Autodesk Fusion 360 part; units mm, degrees
(part 3 of 4)
sketch "Sketch9" plane through (0, 0, 1.5) normal (0, 0, 1) x (-1, 0, 0)
  ellipse E0 centre (-56, -51.25) end of major axis (-52, -51.25) minor radius 1 (-56, -52.25) -> (-56, -50.25) ccw
  line L0 (-56, -52.25) -> (-74.75, -52.25)
  ellipse E1 centre (-74.75, -51.25) end of major axis (-70.75, -51.25) minor radius 1 (-74.75, -50.25) -> (-74.75, -52.25) ccw
  line L1 (-74.75, -50.25) -> (-56, -50.25)
  ellipse E2 centre (-74.75, -23.25) end of major axis (-70.75, -23.25) minor radius 1 (-74.75, -22.25) -> (-74.75, -24.25) ccw
  line L2 (-74.75, -22.25) -> (-56, -22.25)
  ellipse E3 centre (-56, -23.25) end of major axis (-52, -23.25) minor radius 1 (-56, -24.25) -> (-56, -22.25) ccw
  line L3 (-56, -24.25) -> (-74.75, -24.25)
  ellipse E4 centre (-38, -30.25) end of major axis (-34, -30.25) minor radius 1 (-38, -29.25) -> (-38, -31.25) ccw
  line L4 (-38, -29.25) -> (-19.25, -29.25)
  ellipse E5 centre (-19.25, -30.25) end of major axis (-15.25, -30.25) minor radius 1 (-19.25, -31.25) -> (-19.25, -29.25) ccw
  line L5 (-19.25, -31.25) -> (-38, -31.25)
  ellipse E6 centre (-38, -58.25) end of major axis (-34, -58.25) minor radius 1 (-38, -57.25) -> (-38, -59.25) ccw
  line L6 (-38, -57.25) -> (-19.25, -57.25)
  ellipse E7 centre (-19.25, -58.25) end of major axis (-15.25, -58.25) minor radius 1 (-19.25, -59.25) -> (-19.25, -57.25) ccw
  line L7 (-19.25, -59.25) -> (-38, -59.25)
  ellipse E8 centre (-19.25, -51.25) end of major axis (-15.25, -51.25) minor radius 1 (-19.25, -52.25) -> (-19.25, -50.25) ccw
  line L8 (-19.25, -52.25) -> (-38, -52.25)
  ellipse E9 centre (-38, -51.25) end of major axis (-34, -51.25) minor radius 1 (-38, -50.25) -> (-38, -52.25) ccw
  line L9 (-38, -50.25) -> (-19.25, -50.25)
  ellipse E10 centre (-19.25, -23.25) end of major axis (-15.25, -23.25) minor radius 1 (-19.25, -24.25) -> (-19.25, -22.25) ccw
  line L10 (-19.25, -24.25) -> (-38, -24.25)
  ellipse E11 centre (-38, -23.25) end of major axis (-34, -23.25) minor radius 1 (-38, -22.25) -> (-38, -24.25) ccw
  line L11 (-38, -22.25) -> (-19.25, -22.25)
  ellipse E12 centre (-74.75, -30.25) end of major axis (-70.75, -30.25) minor radius 1 (-74.75, -29.25) -> (-74.75, -31.25) ccw
  line L12 (-74.75, -29.25) -> (-56, -29.25)
  ellipse E13 centre (-56, -30.25) end of major axis (-52, -30.25) minor radius 1 (-56, -31.25) -> (-56, -29.25) ccw
  line L13 (-56, -31.25) -> (-74.75, -31.25)
  ellipse E14 centre (-74.75, -58.25) end of major axis (-70.75, -58.25) minor radius 1 (-74.75, -57.25) -> (-74.75, -59.25) ccw
  line L14 (-74.75, -57.25) -> (-56, -57.25)
  ellipse E15 centre (-56, -58.25) end of major axis (-52, -58.25) minor radius 1 (-56, -59.25) -> (-56, -57.25) ccw
  line L15 (-56, -59.25) -> (-74.75, -59.25)
  ellipse E16 centre (-74.75, -44.25) end of major axis (-70.75, -44.25) minor radius 1 (-74.75, -43.25) -> (-74.75, -45.25) ccw
  line L16 (-74.75, -43.25) -> (-56, -43.25)
  ellipse E17 centre (-56, -44.25) end of major axis (-52, -44.25) minor radius 1 (-56, -45.25) -> (-56, -43.25) ccw
  line L17 (-56, -45.25) -> (-74.75, -45.25)
  ellipse E18 centre (-74.75, -16.25) end of major axis (-70.75, -16.25) minor radius 1 (-74.75, -15.25) -> (-74.75, -17.25) ccw
  line L18 (-74.75, -15.25) -> (-56, -15.25)
  ellipse E19 centre (-56, -16.25) end of major axis (-52, -16.25) minor radius 1 (-56, -17.25) -> (-56, -15.25) ccw
  line L19 (-56, -17.25) -> (-74.75, -17.25)
  ellipse E20 centre (-19.25, -37.25) end of major axis (-15.25, -37.25) minor radius 1 (-19.25, -38.25) -> (-19.25, -36.25) ccw
  line L20 (-19.25, -38.25) -> (-38, -38.25)
  ellipse E21 centre (-38, -37.25) end of major axis (-34, -37.25) minor radius 1 (-38, -36.25) -> (-38, -38.25) ccw
  line L21 (-38, -36.25) -> (-19.25, -36.25)
  ellipse E22 centre (-19.25, -65.25) end of major axis (-15.25, -65.25) minor radius 1 (-19.25, -66.25) -> (-19.25, -64.25) ccw
  line L22 (-19.25, -66.25) -> (-38, -66.25)
  ellipse E23 centre (-38, -65.25) end of major axis (-34, -65.25) minor radius 1 (-38, -64.25) -> (-38, -66.25) ccw
  line L23 (-38, -64.25) -> (-19.25, -64.25)
  ellipse E24 centre (-38, -44.25) end of major axis (-34, -44.25) minor radius 1 (-38, -43.25) -> (-38, -45.25) ccw
  line L24 (-38, -43.25) -> (-19.25, -43.25)
  ellipse E25 centre (-19.25, -44.25) end of major axis (-15.25, -44.25) minor radius 1 (-19.25, -45.25) -> (-19.25, -43.25) ccw
  line L25 (-19.25, -45.25) -> (-38, -45.25)
  ellipse E26 centre (-38, -16.25) end of major axis (-34, -16.25) minor radius 1 (-38, -15.25) -> (-38, -17.25) ccw
  line L26 (-38, -15.25) -> (-19.25, -15.25)
  ellipse E27 centre (-19.25, -16.25) end of major axis (-15.25, -16.25) minor radius 1 (-19.25, -17.25) -> (-19.25, -15.25) ccw
  line L27 (-19.25, -17.25) -> (-38, -17.25)
  line L28 (-74.75, -36.25) -> (-56, -36.25)
  ellipse E28 centre (-56, -37.25) end of major axis (-52, -37.25) minor radius 1 (-56, -38.25) -> (-56, -36.25) ccw
  line L29 (-56, -38.25) -> (-74.75, -38.25)
  ellipse E29 centre (-74.75, -37.25) end of major axis (-70.75, -37.25) minor radius 1 (-74.75, -36.25) -> (-74.75, -38.25) ccw
  ellipse E30 centre (-74.75, -65.25) end of major axis (-70.75, -65.25) minor radius 1 (-74.75, -64.25) -> (-74.75, -66.25) ccw
  line L30 (-74.75, -64.25) -> (-56, -64.25)
  ellipse E31 centre (-56, -65.25) end of major axis (-52, -65.25) minor radius 1 (-56, -66.25) -> (-56, -64.25) ccw
  line L31 (-56, -66.25) -> (-74.75, -66.25)
  line L32 (-34.7574, -85.9106) -> (-28.1106, -92.5574)
  ellipse E32 centre (-28.8177, -93.2645) end of major axis (-25.9892, -96.0929) minor radius 1 (-29.5248, -93.9716) -> (-28.1106, -92.5574) ccw
  line L33 (-29.5248, -93.9716) -> (-36.1716, -87.3248)
  ellipse E33 centre (-35.4645, -86.6177) end of major axis (-32.636, -89.4461) minor radius 1 (-34.7574, -85.9106) -> (-36.1716, -87.3248) ccw
  ellipse E34 centre (-73.5355, -93.2645) end of major axis (-70.7071, -90.436) minor radius 1 (-74.2426, -92.5574) -> (-72.8284, -93.9716) ccw
  line L34 (-74.2426, -92.5574) -> (-56.8095, -75.1242)
  ellipse E35 centre (-56.1024, -75.8313) end of major axis (-53.2739, -73.0029) minor radius 1 (-55.3953, -76.5384) -> (-56.8095, -75.1242) ccw
  line L35 (-55.3953, -76.5384) -> (-72.8284, -93.9716)
  ellipse E36 centre (-38.4645, -75.7892) end of major axis (-35.636, -78.6177) minor radius 1 (-37.7574, -75.0821) -> (-39.1716, -76.4963) ccw
  line L36 (-37.7574, -75.0821) -> (-20.2821, -92.5574)
  ellipse E37 centre (-20.9892, -93.2645) end of major axis (-18.1608, -96.0929) minor radius 1 (-21.6963, -93.9716) -> (-20.2821, -92.5574) ccw
  line L37 (-21.6963, -93.9716) -> (-39.1716, -76.4963)
  ellipse E38 centre (-58.5355, -93.9213) end of major axis (-55.7071, -91.0929) minor radius 1 (-57.5048, -94.2952) -> (-58.9094, -92.8906) ccw
  ellipse E39 centre (-57.8787, -93.2645) end of major axis (-55.0503, -90.436) minor radius 1 (-58.9094, -92.8906) -> (-57.5048, -94.2952) ccw
  ellipse E40 centre (-65.7071, -93.2645) end of major axis (-62.8787, -90.436) minor radius 1 (-66.4142, -92.5574) -> (-65, -93.9716) ccw
  line L38 (-66.4142, -92.5574) -> (-59.2426, -85.3858)
  ellipse E41 centre (-58.5355, -86.0929) end of major axis (-55.7071, -83.2645) minor radius 1 (-57.8284, -86.8) -> (-59.2426, -85.3858) ccw
  line L39 (-57.8284, -86.8) -> (-65, -93.9716)
  ellipse E42 centre (-35.6289, -93.7569) end of major axis (-32.8005, -96.5853) minor radius 1 (-35.1707, -92.8062) -> (-36.5796, -94.2151) ccw
  ellipse E43 centre (-36.1213, -93.2645) end of major axis (-33.2929, -96.0929) minor radius 1 (-36.5796, -94.2151) -> (-35.1707, -92.8062) ccw
  line L40 (-93.75, -111.8) -> (-0.25, -111.8)
  line L41 (-0.25, -111.8) -> (-0.25, -0.25)
  line L42 (-0.25, -0.25) -> (-93.75, -0.25)
  line L43 (-93.75, -0.25) -> (-93.75, -111.8)
  circle A0 centre (-5, -5) radius 2
  circle A1 centre (-3.5, -95.55) radius 2
  circle A2 centre (-90.5, -95.55) radius 2
  circle A3 centre (-87.5, -6.5) radius 2
  line L44 (-42.5, -83.8) -> (-42.5, -96.8)
  line L45 (-42.5, -96.8) -> (-51.5, -96.8)
  line L46 (-51.5, -96.8) -> (-51.5, -83.8)
  line L47 (-51.5, -83.8) -> (-42.5, -83.8)
  line L48 (-42, -100.3) -> (-42, -110.3)
  line L49 (-42, -110.3) -> (-43.9689, -110.3)
  line L50 (-43.9689, -110.3) -> (-43.9689, -103.55)
  line L51 (-43.9689, -103.55) -> (-47, -101.8)
  line L52 (-47, -101.8) -> (-50.0311, -103.55)
  line L53 (-50.0311, -103.55) -> (-50.0311, -110.3)
  line L54 (-50.0311, -110.3) -> (-52, -110.3)
  line L55 (-52, -110.3) -> (-52, -100.3)
  line L56 (-52, -100.3) -> (-55, -100.3)
  line L57 (-55, -100.3) -> (-55, -80.3)
  line L58 (-55, -80.3) -> (-52, -80.3)
  line L59 (-52, -80.3) -> (-52, -81.8)
  line L60 (-52, -81.8) -> (-53.5, -81.8)
  line L61 (-53.5, -81.8) -> (-53.5, -98.8)
  line L62 (-53.5, -98.8) -> (-40.5, -98.8)
  line L63 (-40.5, -98.8) -> (-40.5, -81.8)
  line L64 (-40.5, -81.8) -> (-42, -81.8)
  line L65 (-42, -81.8) -> (-42, -80.3)
  line L66 (-42, -80.3) -> (-39, -80.3)
  line L67 (-39, -80.3) -> (-39, -100.3)
  line L68 (-39, -100.3) -> (-42, -100.3)
  line L69 (-0.25, -111.8) -> (-15.25, -111.8)
  line L70 (-15.25, -111.8) -> (-15.25, -96.8)
  line L71 (-15.25, -96.8) -> (-0.25, -96.8)
  line L72 (-0.25, -96.8) -> (-0.25, -111.8)
  line L73 (-93.75, -0.25) -> (-78.75, -0.25)
  line L74 (-78.75, -0.25) -> (-78.75, -15.25)
  line L75 (-78.75, -15.25) -> (-93.75, -15.25)
  line L76 (-93.75, -15.25) -> (-93.75, -0.25)
  line L77 (-15.25, -96.8) -> (-78.75, -96.8)
  line L78 (-78.75, -96.8) -> (-78.75, -15.25)
  line L79 (-78.75, -15.25) -> (-15.25, -15.25)
  line L80 (-15.25, -15.25) -> (-15.25, -96.8)
  line L81 (-47, -96.8) -> (-42, -96.8)
  line L82 (-42, -96.8) -> (-42, -15.25)
  line L83 (-42, -15.25) -> (-47, -15.25)
  line L84 (-47, -15.25) -> (-47, -96.8)
  line L85 (-47, -96.8) -> (-52, -96.8)
  line L86 (-52, -96.8) -> (-52, -15.25)
  line L87 (-52, -15.25) -> (-47, -15.25)
  line L88 (-47, -15.25) -> (-47, -96.8)
  line L89 (-28.625, -66.25) -> (-42, -66.25)
  line L90 (-28.625, -66.25) -> (-15.25, -66.25)
  line L91 (-15.25, -66.25) -> (-78.75, -66.25)
  line L92 (-29.0197, -83.8197) -> (-16.0395, -96.8)
  line L93 (-16.0395, -96.8) -> (-11.0395, -96.8)
  line L94 (-29.2885, -83.551) -> (-29.0197, -83.8197)
  line L95 (-29.0197, -83.8197) -> (-42, -70.8395)
  line L96 (-42, -70.8395) -> (-42, -68.8395)
  line L97 (-42, -68.8395) -> (-15.25, -84.2836)
  line L98 (-42, -68.8395) -> (-11.1118, -68.8395) construction
  line L99 (-42, -68.8395) -> (-41, -67.1074)
  line L100 (-41, -67.1074) -> (-15.25, -81.9742)
  line L101 (-15.25, -81.9742) -> (-16.25, -83.7063)
  line L102 (-16.25, -83.7063) -> (-19.7141, -81.7063)
  line L103 (-19.7141, -81.7063) -> (-18.7141, -79.9742)
  line L104 (-42, -68.8395) -> (-38.5359, -70.8395)
  line L105 (-38.5359, -70.8395) -> (-37.5359, -69.1074)
  line L106 (-42, -68.8395) -> (-52, -68.8395)
  line L107 (-52, -68.8395) -> (-78.75, -84.2836)
  line L108 (-52, -68.8395) -> (-53, -67.1074)
  line L109 (-53, -67.1074) -> (-78.75, -81.9742)
  line L110 (-78.75, -81.9742) -> (-77.75, -83.7063)
  line L111 (-52, -68.8395) -> (-55.4641, -70.8395)
  line L112 (-55.4641, -70.8395) -> (-56.4641, -69.1074)
  line L113 (-55.4641, -70.8395) -> (-53.4641, -70.8395) construction
  line L114 (-77.75, -83.7063) -> (-74.2859, -81.7063)
  line L115 (-74.2859, -81.7063) -> (-75.2859, -79.9742)
  ellipse E44 centre (-19.2141, -80.8402) end of major axis (-19.7141, -81.7063) minor radius 4
  line L116 (-18.7141, -79.9742) -> (-19.7141, -81.7063)
  line L117 (-22.6782, -78.8402) -> (-15.75, -82.8402)
  ellipse E45 centre (-38.0359, -69.9735) end of major axis (-38.5359, -70.8395) minor radius 4
  line L118 (-37.5359, -69.1074) -> (-38.5359, -70.8395)
  line L119 (-41.5, -67.9735) -> (-34.5718, -71.9735)
  ellipse E46 centre (-55.9641, -69.9735) end of major axis (-55.4641, -70.8395) minor radius 4
  line L120 (-56.4641, -69.1074) -> (-55.4641, -70.8395)
  line L121 (-59.4282, -71.9735) -> (-52.5, -67.9735)
  ellipse E47 centre (-74.7859, -80.8402) end of major axis (-74.2859, -81.7063) minor radius 4
  line L122 (-75.2859, -79.9742) -> (-74.2859, -81.7063)
  line L123 (-78.25, -82.8402) -> (-71.3218, -78.8402)
  dimension "d217" = 15
  dimension "d218" = 15
  dimension "d219" = 15
  dimension "d220" = 15
  dimension "d221" = 5
  dimension "d222" = 5
  dimension "d223" = 5
  dimension "d224" = 2
  dimension "d225" = 30
  dimension "d226" = 2
  dimension "d227" = 4
  dimension "d228" = 4
  dimension "d229" = 30
  dimension "d230" = 90
  dimension "d231" = 2
  dimension "d232" = 4
  dimension "d233" = 120
  dimension "d234" = 4
  constraint horizontal L69
  constraint vertical L70
  constraint horizontal L71
  constraint vertical L72
  constraint coincident L40.end L41.start
  constraint horizontal L73
  constraint vertical L74
  constraint horizontal L75
  constraint vertical L76
  constraint coincident L42.end L43.start
  constraint horizontal L77
  constraint vertical L78
  constraint horizontal L79
  constraint vertical L80
  constraint horizontal L81
  constraint vertical L82
  constraint horizontal L83
  constraint vertical L84
  constraint coincident L79 L82.end
  constraint midpoint L45 L81.start
  constraint horizontal L85
  constraint vertical L86
  constraint horizontal L87
  constraint vertical L88
  constraint midpoint L22 L89.start
  constraint coincident L82 L89.end
  constraint perpendicular L82 L89
  constraint coincident L80 L90.end
  constraint perpendicular L80 L90
  constraint coincident L78 L91.end
  constraint perpendicular L78 L91
  constraint midpoint L36 L92.start
  constraint coincident L77 L92.end
  constraint parallel L36 L92
  constraint perpendicular L70 L93
  constraint coincident L36 L94.start
  constraint parallel L92 L94
  constraint coincident L82 L95.end
  constraint parallel L36 L95
  constraint parallel L82 L96
  constraint horizontal L98
  constraint coincident L80 L97.end
  constraint perpendicular L97 L99
  constraint coincident L80 L100.end
  constraint perpendicular L99 L100
  constraint coincident L97 L101.end
  constraint perpendicular L97 L101
  constraint perpendicular L101 L102
  constraint coincident L100 L103.end
  constraint perpendicular L100 L103
  constraint perpendicular L99 L104
  constraint coincident L100 L105.end
  constraint perpendicular L100 L105
  constraint coincident L86 L106.end
  constraint perpendicular L86 L106
  constraint coincident L78 L107.end
  constraint coincident L78 L109.end
  constraint perpendicular L108 L109
  constraint coincident L107 L110.end
  constraint perpendicular L107 L110
  constraint perpendicular L110 L111
  constraint horizontal L113
  constraint coincident L109 L112.end
  constraint perpendicular L110 L114
  constraint coincident L109 L115.end
  constraint perpendicular L109 L115
  constraint midpoint L103 E44.centre
  constraint coincident L103.end E44
  constraint coincident L102.end E44
  constraint midpoint L105 E45.centre
  constraint coincident L105.end E45
  constraint coincident L104.end E45
  constraint midpoint L112 E46.centre
  constraint coincident L112.end E46
  constraint coincident L111.end E46
  constraint midpoint L115 E47.centre
  constraint coincident L115.end E47
  constraint coincident L114.end E47
  measures "d217" distance of L40.end L69.end
  measures "d218" distance of L40.end L71.end
  measures "d219" distance of L42.end L73.end
  measures "d220" distance of L42.end L75.end
  measures "d221" distance of L81.start L81.end
  measures "d222" distance of L81.start L85.end
  measures "d223" distance of L92.end L93.end
  measures "d224" distance of L95.end L96.end
  measures "d225" angle of L97 L98
  measures "d226" distance of L96.end L99.end
  measures "d227" distance of L101.end L102.end
  measures "d228" distance of L96.end L104.end
  measures "d229" angle of L106 L107
  measures "d230" angle of L107 L108
  measures "d231" distance of L106.end L108.end
  measures "d232" distance of L106.end L111.end
  measures "d233" angle of L112 L113
  measures "d234" distance of L110.end L114.end
extrude "Extrude13" cut sketch "Sketch9" against normal blind 4 contours L112 E46 L120 L121 | L107 L109 E46 E47 | L112 E46 L120 L121 | L112 E46 L120 L121 | L115 E47 L122 L123 | L115 E47 L122 L123 | L112 E46 L120 L121 | L115 E47 L122 L123 | L115 E47 L122 L123 | L97 L100 E44 E45 | L105 E45 L118 L119 | L105 E45 L118 L119 | L105 E45 L118 L119 | L103 E44 L116 L117 | L103 E44 L116 L117 | L105 E45 L118 L119 | L103 E44 L116 L117 | L103 E44 L116 L117
sketch "Sketch10" plane through (0, 0, 1.5) normal (0, 0, 1) x (-1, 0, 0)
  ellipse E0 centre (-19.2141, -80.8402) end of major axis (-15.75, -82.8402) minor radius 1 (-19.7141, -81.7063) -> (-18.7141, -79.9742) ccw
  line L0 (-19.7141, -81.7063) -> (-38.5359, -70.8395)
  ellipse E1 centre (-38.0359, -69.9735) end of major axis (-34.5718, -71.9735) minor radius 1 (-37.5359, -69.1074) -> (-38.5359, -70.8395) ccw
  line L1 (-37.5359, -69.1074) -> (-18.7141, -79.9742)
  ellipse E2 centre (-74.7859, -80.8402) end of major axis (-71.3218, -78.8402) minor radius 1 (-75.2859, -79.9742) -> (-74.2859, -81.7063) ccw
  line L2 (-75.2859, -79.9742) -> (-56.4641, -69.1074)
  ellipse E3 centre (-55.9641, -69.9735) end of major axis (-52.5, -67.9735) minor radius 1 (-55.4641, -70.8395) -> (-56.4641, -69.1074) ccw
  line L3 (-55.4641, -70.8395) -> (-74.2859, -81.7063)
  ellipse E4 centre (-56, -51.25) end of major axis (-52, -51.25) minor radius 1 (-56, -52.25) -> (-56, -50.25) ccw
  line L4 (-56, -52.25) -> (-74.75, -52.25)
  ellipse E5 centre (-74.75, -51.25) end of major axis (-70.75, -51.25) minor radius 1 (-74.75, -50.25) -> (-74.75, -52.25) ccw
  line L5 (-74.75, -50.25) -> (-56, -50.25)
  ellipse E6 centre (-74.75, -23.25) end of major axis (-70.75, -23.25) minor radius 1 (-74.75, -22.25) -> (-74.75, -24.25) ccw
  line L6 (-74.75, -22.25) -> (-56, -22.25)
  ellipse E7 centre (-56, -23.25) end of major axis (-52, -23.25) minor radius 1 (-56, -24.25) -> (-56, -22.25) ccw
  line L7 (-56, -24.25) -> (-74.75, -24.25)
  ellipse E8 centre (-38, -30.25) end of major axis (-34, -30.25) minor radius 1 (-38, -29.25) -> (-38, -31.25) ccw
  line L8 (-38, -29.25) -> (-19.25, -29.25)
  ellipse E9 centre (-19.25, -30.25) end of major axis (-15.25, -30.25) minor radius 1 (-19.25, -31.25) -> (-19.25, -29.25) ccw
  line L9 (-19.25, -31.25) -> (-38, -31.25)
  ellipse E10 centre (-38, -58.25) end of major axis (-34, -58.25) minor radius 1 (-38, -57.25) -> (-38, -59.25) ccw
  line L10 (-38, -57.25) -> (-19.25, -57.25)
  ellipse E11 centre (-19.25, -58.25) end of major axis (-15.25, -58.25) minor radius 1 (-19.25, -59.25) -> (-19.25, -57.25) ccw
  line L11 (-19.25, -59.25) -> (-38, -59.25)
  ellipse E12 centre (-19.25, -51.25) end of major axis (-15.25, -51.25) minor radius 1 (-19.25, -52.25) -> (-19.25, -50.25) ccw
  line L12 (-19.25, -52.25) -> (-38, -52.25)
  ellipse E13 centre (-38, -51.25) end of major axis (-34, -51.25) minor radius 1 (-38, -50.25) -> (-38, -52.25) ccw
  line L13 (-38, -50.25) -> (-19.25, -50.25)
  ellipse E14 centre (-19.25, -23.25) end of major axis (-15.25, -23.25) minor radius 1 (-19.25, -24.25) -> (-19.25, -22.25) ccw
  line L14 (-19.25, -24.25) -> (-38, -24.25)
  ellipse E15 centre (-38, -23.25) end of major axis (-34, -23.25) minor radius 1 (-38, -22.25) -> (-38, -24.25) ccw
  line L15 (-38, -22.25) -> (-19.25, -22.25)
  ellipse E16 centre (-74.75, -30.25) end of major axis (-70.75, -30.25) minor radius 1 (-74.75, -29.25) -> (-74.75, -31.25) ccw
  line L16 (-74.75, -29.25) -> (-56, -29.25)
  ellipse E17 centre (-56, -30.25) end of major axis (-52, -30.25) minor radius 1 (-56, -31.25) -> (-56, -29.25) ccw
  line L17 (-56, -31.25) -> (-74.75, -31.25)
  ellipse E18 centre (-74.75, -58.25) end of major axis (-70.75, -58.25) minor radius 1 (-74.75, -57.25) -> (-74.75, -59.25) ccw
  line L18 (-74.75, -57.25) -> (-56, -57.25)
  ellipse E19 centre (-56, -58.25) end of major axis (-52, -58.25) minor radius 1 (-56, -59.25) -> (-56, -57.25) ccw
  line L19 (-56, -59.25) -> (-74.75, -59.25)
  ellipse E20 centre (-74.75, -44.25) end of major axis (-70.75, -44.25) minor radius 1 (-74.75, -43.25) -> (-74.75, -45.25) ccw
  line L20 (-74.75, -43.25) -> (-56, -43.25)
  ellipse E21 centre (-56, -44.25) end of major axis (-52, -44.25) minor radius 1 (-56, -45.25) -> (-56, -43.25) ccw
  line L21 (-56, -45.25) -> (-74.75, -45.25)
  ellipse E22 centre (-74.75, -16.25) end of major axis (-70.75, -16.25) minor radius 1 (-74.75, -15.25) -> (-74.75, -17.25) ccw
  line L22 (-74.75, -15.25) -> (-56, -15.25)
  ellipse E23 centre (-56, -16.25) end of major axis (-52, -16.25) minor radius 1 (-56, -17.25) -> (-56, -15.25) ccw
  line L23 (-56, -17.25) -> (-74.75, -17.25)
  ellipse E24 centre (-19.25, -37.25) end of major axis (-15.25, -37.25) minor radius 1 (-19.25, -38.25) -> (-19.25, -36.25) ccw
  line L24 (-19.25, -38.25) -> (-38, -38.25)
  ellipse E25 centre (-38, -37.25) end of major axis (-34, -37.25) minor radius 1 (-38, -36.25) -> (-38, -38.25) ccw
  line L25 (-38, -36.25) -> (-19.25, -36.25)
  ellipse E26 centre (-19.25, -65.25) end of major axis (-15.25, -65.25) minor radius 1 (-19.25, -66.25) -> (-19.25, -64.25) ccw
  line L26 (-19.25, -66.25) -> (-38, -66.25)
  ellipse E27 centre (-38, -65.25) end of major axis (-34, -65.25) minor radius 1 (-38, -64.25) -> (-38, -66.25) ccw
  line L27 (-38, -64.25) -> (-19.25, -64.25)
  ellipse E28 centre (-38, -44.25) end of major axis (-34, -44.25) minor radius 1 (-38, -43.25) -> (-38, -45.25) ccw
  line L28 (-38, -43.25) -> (-19.25, -43.25)
  ellipse E29 centre (-19.25, -44.25) end of major axis (-15.25, -44.25) minor radius 1 (-19.25, -45.25) -> (-19.25, -43.25) ccw
  line L29 (-19.25, -45.25) -> (-38, -45.25)
  ellipse E30 centre (-38, -16.25) end of major axis (-34, -16.25) minor radius 1 (-38, -15.25) -> (-38, -17.25) ccw
  line L30 (-38, -15.25) -> (-19.25, -15.25)
  ellipse E31 centre (-19.25, -16.25) end of major axis (-15.25, -16.25) minor radius 1 (-19.25, -17.25) -> (-19.25, -15.25) ccw
  line L31 (-19.25, -17.25) -> (-38, -17.25)
  line L32 (-74.75, -36.25) -> (-56, -36.25)
  ellipse E32 centre (-56, -37.25) end of major axis (-52, -37.25) minor radius 1 (-56, -38.25) -> (-56, -36.25) ccw
  line L33 (-56, -38.25) -> (-74.75, -38.25)
  ellipse E33 centre (-74.75, -37.25) end of major axis (-70.75, -37.25) minor radius 1 (-74.75, -36.25) -> (-74.75, -38.25) ccw
  ellipse E34 centre (-74.75, -65.25) end of major axis (-70.75, -65.25) minor radius 1 (-74.75, -64.25) -> (-74.75, -66.25) ccw
  line L34 (-74.75, -64.25) -> (-56, -64.25)
  ellipse E35 centre (-56, -65.25) end of major axis (-52, -65.25) minor radius 1 (-56, -66.25) -> (-56, -64.25) ccw
  line L35 (-56, -66.25) -> (-74.75, -66.25)
  line L36 (-34.7574, -85.9106) -> (-28.1106, -92.5574)
  ellipse E36 centre (-28.8177, -93.2645) end of major axis (-25.9892, -96.0929) minor radius 1 (-29.5248, -93.9716) -> (-28.1106, -92.5574) ccw
  line L37 (-29.5248, -93.9716) -> (-36.1716, -87.3248)
  ellipse E37 centre (-35.4645, -86.6177) end of major axis (-32.636, -89.4461) minor radius 1 (-34.7574, -85.9106) -> (-36.1716, -87.3248) ccw
  ellipse E38 centre (-73.5355, -93.2645) end of major axis (-70.7071, -90.436) minor radius 1 (-74.2426, -92.5574) -> (-72.8284, -93.9716) ccw
  line L38 (-74.2426, -92.5574) -> (-56.8095, -75.1242)
  ellipse E39 centre (-56.1024, -75.8313) end of major axis (-53.2739, -73.0029) minor radius 1 (-55.3953, -76.5384) -> (-56.8095, -75.1242) ccw
  line L39 (-55.3953, -76.5384) -> (-72.8284, -93.9716)
  ellipse E40 centre (-38.4645, -75.7892) end of major axis (-35.636, -78.6177) minor radius 1 (-37.7574, -75.0821) -> (-39.1716, -76.4963) ccw
  line L40 (-37.7574, -75.0821) -> (-20.2821, -92.5574)
  ellipse E41 centre (-20.9892, -93.2645) end of major axis (-18.1608, -96.0929) minor radius 1 (-21.6963, -93.9716) -> (-20.2821, -92.5574) ccw
  line L41 (-21.6963, -93.9716) -> (-39.1716, -76.4963)
  ellipse E42 centre (-58.5355, -93.9213) end of major axis (-55.7071, -91.0929) minor radius 1 (-57.5048, -94.2952) -> (-58.9094, -92.8906) ccw
  ellipse E43 centre (-57.8787, -93.2645) end of major axis (-55.0503, -90.436) minor radius 1 (-58.9094, -92.8906) -> (-57.5048, -94.2952) ccw
  ellipse E44 centre (-65.7071, -93.2645) end of major axis (-62.8787, -90.436) minor radius 1 (-66.4142, -92.5574) -> (-65, -93.9716) ccw
  line L42 (-66.4142, -92.5574) -> (-59.2426, -85.3858)
  ellipse E45 centre (-58.5355, -86.0929) end of major axis (-55.7071, -83.2645) minor radius 1 (-57.8284, -86.8) -> (-59.2426, -85.3858) ccw
  line L43 (-57.8284, -86.8) -> (-65, -93.9716)
  ellipse E46 centre (-35.6289, -93.7569) end of major axis (-32.8005, -96.5853) minor radius 1 (-35.1707, -92.8062) -> (-36.5796, -94.2151) ccw
  ellipse E47 centre (-36.1213, -93.2645) end of major axis (-33.2929, -96.0929) minor radius 1 (-36.5796, -94.2151) -> (-35.1707, -92.8062) ccw
  line L44 (-93.75, -111.8) -> (-0.25, -111.8)
  line L45 (-0.25, -111.8) -> (-0.25, -0.25)
  line L46 (-0.25, -0.25) -> (-93.75, -0.25)
  line L47 (-93.75, -0.25) -> (-93.75, -111.8)
  circle A0 centre (-5, -5) radius 2
  circle A1 centre (-3.5, -95.55) radius 2
  circle A2 centre (-90.5, -95.55) radius 2
  circle A3 centre (-87.5, -6.5) radius 2
  line L48 (-42.5, -83.8) -> (-42.5, -96.8)
  line L49 (-42.5, -96.8) -> (-51.5, -96.8)
  line L50 (-51.5, -96.8) -> (-51.5, -83.8)
  line L51 (-51.5, -83.8) -> (-42.5, -83.8)
  line L52 (-42, -100.3) -> (-42, -110.3)
  line L53 (-42, -110.3) -> (-43.9689, -110.3)
  line L54 (-43.9689, -110.3) -> (-43.9689, -103.55)
  line L55 (-43.9689, -103.55) -> (-47, -101.8)
  line L56 (-47, -101.8) -> (-50.0311, -103.55)
  line L57 (-50.0311, -103.55) -> (-50.0311, -110.3)
  line L58 (-50.0311, -110.3) -> (-52, -110.3)
  line L59 (-52, -110.3) -> (-52, -100.3)
  line L60 (-52, -100.3) -> (-55, -100.3)
  line L61 (-55, -100.3) -> (-55, -80.3)
  line L62 (-55, -80.3) -> (-52, -80.3)
  line L63 (-52, -80.3) -> (-52, -81.8)
  line L64 (-52, -81.8) -> (-53.5, -81.8)
  line L65 (-53.5, -81.8) -> (-53.5, -98.8)
  line L66 (-53.5, -98.8) -> (-40.5, -98.8)
  line L67 (-40.5, -98.8) -> (-40.5, -81.8)
  line L68 (-40.5, -81.8) -> (-42, -81.8)
  line L69 (-42, -81.8) -> (-42, -80.3)
  line L70 (-42, -80.3) -> (-39, -80.3)
  line L71 (-39, -80.3) -> (-39, -100.3)
  line L72 (-39, -100.3) -> (-42, -100.3)
  line L73 (-0.25, -111.8) -> (-15.25, -111.8)
  line L74 (-15.25, -111.8) -> (-15.25, -96.8)
  line L75 (-15.25, -96.8) -> (-0.25, -96.8)
  line L76 (-0.25, -96.8) -> (-0.25, -111.8)
  line L77 (-93.75, -0.25) -> (-78.75, -0.25)
  line L78 (-78.75, -0.25) -> (-78.75, -15.25)
  line L79 (-78.75, -15.25) -> (-93.75, -15.25)
  line L80 (-93.75, -15.25) -> (-93.75, -0.25)
  line L81 (-78.75, -15.25) -> (-15.25, -15.25)
  line L82 (-15.25, -15.25) -> (-15.25, -96.8)
  line L83 (-15.25, -96.8) -> (-78.75, -96.8)
  line L84 (-78.75, -96.8) -> (-78.75, -15.25)
  line L85 (-47, -96.8) -> (-42, -96.8)
  line L86 (-42, -96.8) -> (-42, -47.714)
  line L87 (-42, -47.714) -> (-47, -47.714)
  line L88 (-47, -47.714) -> (-47, -96.8)
  line L89 (-47, -96.8) -> (-52, -96.8)
  line L90 (-52, -96.8) -> (-52, -48)
  line L91 (-52, -48) -> (-47, -48)
  line L92 (-47, -48) -> (-47, -96.8)
  line L93 (-28.125, -74.5408) -> (-42, -66.5301)
  line L94 (-42, -66.5301) -> (-15.25, -73.6977)
  line L95 (-42, -66.5301) -> (-32.3407, -69.1183)
  line L96 (-32.3407, -69.1183) -> (-31.8231, -67.1864)
  line L97 (-32.3407, -69.1183) -> (-30.3407, -69.1183) construction
  line L98 (-31.8231, -67.1864) -> (-15.25, -71.6272)
  line L99 (-31.8231, -67.1864) -> (-14.6654, -67.1864) construction
  line L100 (-15.25, -71.6272) -> (-15.7676, -73.559)
  line L101 (-15.7676, -73.559) -> (-19.6313, -72.5237)
  line L102 (-19.6313, -72.5237) -> (-19.1137, -70.5919)
  line L103 (-32.3407, -69.1183) -> (-28.477, -70.1535)
  line L104 (-28.477, -70.1535) -> (-27.9594, -68.2217)
  line L105 (-42, -66.5301) -> (-52, -66.5301)
  line L106 (-52, -66.5301) -> (-78.75, -73.6977)
  line L107 (-52, -66.5301) -> (-61.6593, -69.1183)
  line L108 (-61.6593, -69.1183) -> (-62.1769, -67.1864)
  line L109 (-62.1769, -67.1864) -> (-78.75, -71.6272)
  line L110 (-78.75, -71.6272) -> (-78.2324, -73.559)
  line L111 (-61.6593, -69.1183) -> (-65.523, -70.1535)
  line L112 (-78.2324, -73.559) -> (-74.3687, -72.5237)
  line L113 (-65.523, -70.1535) -> (-66.0406, -68.2217)
  line L114 (-74.3687, -72.5237) -> (-74.8863, -70.5919)
  ellipse E48 centre (-19.3725, -71.5578) end of major axis (-19.6313, -72.5237) minor radius 4
  line L115 (-19.1137, -70.5919) -> (-19.6313, -72.5237)
  line L116 (-23.2362, -70.5225) -> (-15.5088, -72.5931)
  ellipse E49 centre (-28.2182, -69.1876) end of major axis (-28.477, -70.1535) minor radius 4.0176
  line L117 (-27.9594, -68.2217) -> (-28.477, -70.1535)
  line L118 (-32.099, -68.1478) -> (-24.3375, -70.2275)
  ellipse E50 centre (-65.7818, -69.1876) end of major axis (-65.523, -70.1535) minor radius 4
  line L119 (-66.0406, -68.2217) -> (-65.523, -70.1535)
  line L120 (-69.6455, -70.2229) -> (-61.9181, -68.1523)
  ellipse E51 centre (-74.6275, -71.5578) end of major axis (-74.3687, -72.5237) minor radius 4
  line L121 (-74.8863, -70.5919) -> (-74.3687, -72.5237)
  line L122 (-78.4912, -72.5931) -> (-70.7638, -70.5225)
  dimension "d237" = 15
  dimension "d238" = 15
  dimension "d239" = 15
  dimension "d240" = 15
  dimension "d241" = 5
  dimension "d242" = 15
  dimension "d243" = 10
  dimension "d244" = 75
  dimension "d245" = 2
  dimension "d246" = 15
  dimension "d247" = 4
  dimension "d248" = 4
  dimension "d249" = 15
  dimension "d250" = 10
  dimension "d251" = 2
  dimension "d252" = 2
  dimension "d253" = 4
  dimension "d254" = 4
  constraint horizontal L73
  constraint vertical L74
  constraint horizontal L75
  constraint vertical L76
  constraint coincident L44.end L45.start
  constraint horizontal L77
  constraint vertical L78
  constraint horizontal L79
  constraint vertical L80
  constraint coincident L46.end L47.start
  constraint horizontal L81
  constraint vertical L82
  constraint horizontal L83
  constraint vertical L84
  constraint horizontal L85
  constraint vertical L86
  constraint horizontal L87
  constraint vertical L88
  constraint midpoint L83 L85.start
  constraint horizontal L89
  constraint vertical L90
  constraint horizontal L91
  constraint vertical L92
  constraint midpoint L1 L93.start
  constraint coincident L86 L93.end
  constraint parallel L1 L93
  constraint coincident L82 L94.end
  constraint parallel L94 L95
  constraint horizontal L97
  constraint horizontal L99
  constraint coincident L82 L98.end
  constraint coincident L94 L100.end
  constraint perpendicular L94 L100
  constraint perpendicular L100 L101
  constraint coincident L98 L102.end
  constraint perpendicular L98 L102
  constraint perpendicular L96 L103
  constraint coincident L98 L104.end
  constraint perpendicular L98 L104
  constraint coincident L90 L105.end
  constraint perpendicular L90 L105
  constraint coincident L84 L106.end
  constraint parallel L106 L107
  constraint perpendicular L106 L108
  constraint coincident L84 L109.end
  constraint perpendicular L108 L109
  constraint coincident L106 L110.end
  constraint perpendicular L106 L110
  constraint perpendicular L108 L111
  constraint perpendicular L110 L112
  constraint coincident L109 L113.end
  constraint perpendicular L109 L113
  constraint coincident L109 L114.end
  constraint perpendicular L109 L114
  constraint midpoint L102 E48.centre
  constraint coincident L102.end E48
  constraint coincident L101.end E48
  constraint midpoint L104 E49.centre
  constraint coincident L104.end E49
  constraint coincident L103.end E49
  constraint midpoint L113 E50.centre
  constraint coincident L113.end E50
  constraint coincident L111.end E50
  constraint midpoint L114 E51.centre
  constraint coincident L114.end E51
  constraint coincident L112.end E51
  measures "d237" distance of L44.end L73.end
  measures "d238" distance of L44.end L75.end
  measures "d239" distance of L46.end L77.end
  measures "d240" distance of L46.end L79.end
  measures "d241" distance of L85.start L85.end
  measures "d242" angle of L93 L94
  measures "d243" distance of L93.end L95.end
  measures "d244" angle of L96 L97
  measures "d245" distance of L95.end L96.end
  measures "d246" angle of L98 L99
  measures "d247" distance of L100.end L101.end
  measures "d248" distance of L95.end L103.end
  measures "d249" angle of L105 L106
  measures "d250" distance of L105.end L107.end
  measures "d251" distance of L107.end L108.end
  measures "d252" distance of L109.end L110.end
  measures "d253" distance of L107.end L111.end
  measures "d254" distance of L110.end L112.end
extrude "Extrude14" cut sketch "Sketch10" against normal blind 6 contours L113 E50 L119 L120 | L106 L109 E50 E51 | L113 E50 L119 L120 | L113 E50 L119 L120 | L114 E51 L121 L122 | L114 E51 L121 L122 | L114 E51 L121 L122 | L114 E51 L121 L122 | L113 E50 L119 L120 | L94 L98 E48 E49 | L96 L104 E49 L117 L118 | L104 E49 L117 L118 | L102 E48 L115 L116 | L102 E48 L115 L116 | L96 L104 E49 L117 L118 | L104 E49 L117 L118 | L102 E48 L115 L116 | L102 E48 L115 L116
sketch "Sketch11" plane through (0, 0, 1.5) normal (0, 0, 1) x (-1, 0, 0)
  ellipse E0 centre (-19.3725, -71.5578) end of major axis (-15.5088, -72.5931) minor radius 1 (-19.6313, -72.5237) -> (-19.1137, -70.5919) ccw
  line L0 (-19.6313, -72.5237) -> (-28.477, -70.1535)
  ellipse E1 centre (-28.2182, -69.1876) end of major axis (-24.3375, -70.2275) minor radius 1 (-32.1062, -68.2428) -> (-28.477, -70.1535) ccw
  line L1 (-32.1062, -68.2428) -> (-32.0577, -68.0619)
  ellipse E2 centre (-28.2182, -69.1876) end of major axis (-24.3375, -70.2275) minor radius 1 (-27.9594, -68.2217) -> (-32.0577, -68.0619) ccw
  line L2 (-27.9594, -68.2217) -> (-19.1137, -70.5919)
  ellipse E3 centre (-74.6275, -71.5578) end of major axis (-70.7638, -70.5225) minor radius 1 (-74.8863, -70.5919) -> (-74.3687, -72.5237) ccw
  line L3 (-74.8863, -70.5919) -> (-66.0406, -68.2217)
  ellipse E4 centre (-65.7818, -69.1876) end of major axis (-61.9181, -68.1523) minor radius 1 (-65.523, -70.1535) -> (-66.0406, -68.2217) ccw
  line L4 (-65.523, -70.1535) -> (-74.3687, -72.5237)
  ellipse E5 centre (-19.2141, -80.8402) end of major axis (-15.75, -82.8402) minor radius 1 (-19.7141, -81.7063) -> (-18.7141, -79.9742) ccw
  line L5 (-19.7141, -81.7063) -> (-38.5359, -70.8395)
  ellipse E6 centre (-38.0359, -69.9735) end of major axis (-34.5718, -71.9735) minor radius 1 (-37.5359, -69.1074) -> (-38.5359, -70.8395) ccw
  line L6 (-37.5359, -69.1074) -> (-18.7141, -79.9742)
  ellipse E7 centre (-74.7859, -80.8402) end of major axis (-71.3218, -78.8402) minor radius 1 (-75.2859, -79.9742) -> (-74.2859, -81.7063) ccw
  line L7 (-75.2859, -79.9742) -> (-56.4641, -69.1074)
  ellipse E8 centre (-55.9641, -69.9735) end of major axis (-52.5, -67.9735) minor radius 1 (-55.4641, -70.8395) -> (-56.4641, -69.1074) ccw
  line L8 (-55.4641, -70.8395) -> (-74.2859, -81.7063)
  ellipse E9 centre (-56, -51.25) end of major axis (-52, -51.25) minor radius 1 (-56, -52.25) -> (-56, -50.25) ccw
  line L9 (-56, -52.25) -> (-74.75, -52.25)
  ellipse E10 centre (-74.75, -51.25) end of major axis (-70.75, -51.25) minor radius 1 (-74.75, -50.25) -> (-74.75, -52.25) ccw
  line L10 (-74.75, -50.25) -> (-56, -50.25)
  ellipse E11 centre (-74.75, -23.25) end of major axis (-70.75, -23.25) minor radius 1 (-74.75, -22.25) -> (-74.75, -24.25) ccw
  line L11 (-74.75, -22.25) -> (-56, -22.25)
  ellipse E12 centre (-56, -23.25) end of major axis (-52, -23.25) minor radius 1 (-56, -24.25) -> (-56, -22.25) ccw
  line L12 (-56, -24.25) -> (-74.75, -24.25)
  ellipse E13 centre (-38, -30.25) end of major axis (-34, -30.25) minor radius 1 (-38, -29.25) -> (-38, -31.25) ccw
  line L13 (-38, -29.25) -> (-19.25, -29.25)
  ellipse E14 centre (-19.25, -30.25) end of major axis (-15.25, -30.25) minor radius 1 (-19.25, -31.25) -> (-19.25, -29.25) ccw
  line L14 (-19.25, -31.25) -> (-38, -31.25)
  ellipse E15 centre (-38, -58.25) end of major axis (-34, -58.25) minor radius 1 (-38, -57.25) -> (-38, -59.25) ccw
  line L15 (-38, -57.25) -> (-19.25, -57.25)
  ellipse E16 centre (-19.25, -58.25) end of major axis (-15.25, -58.25) minor radius 1 (-19.25, -59.25) -> (-19.25, -57.25) ccw
  line L16 (-19.25, -59.25) -> (-38, -59.25)
  ellipse E17 centre (-19.25, -51.25) end of major axis (-15.25, -51.25) minor radius 1 (-19.25, -52.25) -> (-19.25, -50.25) ccw
  line L17 (-19.25, -52.25) -> (-38, -52.25)
  ellipse E18 centre (-38, -51.25) end of major axis (-34, -51.25) minor radius 1 (-38, -50.25) -> (-38, -52.25) ccw
  line L18 (-38, -50.25) -> (-19.25, -50.25)
  ellipse E19 centre (-19.25, -23.25) end of major axis (-15.25, -23.25) minor radius 1 (-19.25, -24.25) -> (-19.25, -22.25) ccw
  line L19 (-19.25, -24.25) -> (-38, -24.25)
  ellipse E20 centre (-38, -23.25) end of major axis (-34, -23.25) minor radius 1 (-38, -22.25) -> (-38, -24.25) ccw
  line L20 (-38, -22.25) -> (-19.25, -22.25)
  ellipse E21 centre (-74.75, -30.25) end of major axis (-70.75, -30.25) minor radius 1 (-74.75, -29.25) -> (-74.75, -31.25) ccw
  line L21 (-74.75, -29.25) -> (-56, -29.25)
  ellipse E22 centre (-56, -30.25) end of major axis (-52, -30.25) minor radius 1 (-56, -31.25) -> (-56, -29.25) ccw
  line L22 (-56, -31.25) -> (-74.75, -31.25)
  ellipse E23 centre (-74.75, -58.25) end of major axis (-70.75, -58.25) minor radius 1 (-74.75, -57.25) -> (-74.75, -59.25) ccw
  line L23 (-74.75, -57.25) -> (-56, -57.25)
  ellipse E24 centre (-56, -58.25) end of major axis (-52, -58.25) minor radius 1 (-56, -59.25) -> (-56, -57.25) ccw
  line L24 (-56, -59.25) -> (-74.75, -59.25)
  ellipse E25 centre (-74.75, -44.25) end of major axis (-70.75, -44.25) minor radius 1 (-74.75, -43.25) -> (-74.75, -45.25) ccw
  line L25 (-74.75, -43.25) -> (-56, -43.25)
  ellipse E26 centre (-56, -44.25) end of major axis (-52, -44.25) minor radius 1 (-56, -45.25) -> (-56, -43.25) ccw
  line L26 (-56, -45.25) -> (-74.75, -45.25)
  ellipse E27 centre (-74.75, -16.25) end of major axis (-70.75, -16.25) minor radius 1 (-74.75, -15.25) -> (-74.75, -17.25) ccw
  line L27 (-74.75, -15.25) -> (-56, -15.25)
  ellipse E28 centre (-56, -16.25) end of major axis (-52, -16.25) minor radius 1 (-56, -17.25) -> (-56, -15.25) ccw
  line L28 (-56, -17.25) -> (-74.75, -17.25)
  ellipse E29 centre (-19.25, -37.25) end of major axis (-15.25, -37.25) minor radius 1 (-19.25, -38.25) -> (-19.25, -36.25) ccw
  line L29 (-19.25, -38.25) -> (-38, -38.25)
  ellipse E30 centre (-38, -37.25) end of major axis (-34, -37.25) minor radius 1 (-38, -36.25) -> (-38, -38.25) ccw
  line L30 (-38, -36.25) -> (-19.25, -36.25)
  ellipse E31 centre (-19.25, -65.25) end of major axis (-15.25, -65.25) minor radius 1 (-19.25, -66.25) -> (-19.25, -64.25) ccw
  line L31 (-19.25, -66.25) -> (-38, -66.25)
  ellipse E32 centre (-38, -65.25) end of major axis (-34, -65.25) minor radius 1 (-38, -64.25) -> (-38, -66.25) ccw
  line L32 (-38, -64.25) -> (-19.25, -64.25)
  ellipse E33 centre (-38, -44.25) end of major axis (-34, -44.25) minor radius 1 (-38, -43.25) -> (-38, -45.25) ccw
  line L33 (-38, -43.25) -> (-19.25, -43.25)
  ellipse E34 centre (-19.25, -44.25) end of major axis (-15.25, -44.25) minor radius 1 (-19.25, -45.25) -> (-19.25, -43.25) ccw
  line L34 (-19.25, -45.25) -> (-38, -45.25)
  ellipse E35 centre (-38, -16.25) end of major axis (-34, -16.25) minor radius 1 (-38, -15.25) -> (-38, -17.25) ccw
  line L35 (-38, -15.25) -> (-19.25, -15.25)
  ellipse E36 centre (-19.25, -16.25) end of major axis (-15.25, -16.25) minor radius 1 (-19.25, -17.25) -> (-19.25, -15.25) ccw
  line L36 (-19.25, -17.25) -> (-38, -17.25)
  line L37 (-74.75, -36.25) -> (-56, -36.25)
  ellipse E37 centre (-56, -37.25) end of major axis (-52, -37.25) minor radius 1 (-56, -38.25) -> (-56, -36.25) ccw
  line L38 (-56, -38.25) -> (-74.75, -38.25)
  ellipse E38 centre (-74.75, -37.25) end of major axis (-70.75, -37.25) minor radius 1 (-74.75, -36.25) -> (-74.75, -38.25) ccw
  ellipse E39 centre (-74.75, -65.25) end of major axis (-70.75, -65.25) minor radius 1 (-74.75, -64.25) -> (-74.75, -66.25) ccw
  line L39 (-74.75, -64.25) -> (-56, -64.25)
  ellipse E40 centre (-56, -65.25) end of major axis (-52, -65.25) minor radius 1 (-56, -66.25) -> (-56, -64.25) ccw
  line L40 (-56, -66.25) -> (-74.75, -66.25)
  line L41 (-34.7574, -85.9106) -> (-28.1106, -92.5574)
  ellipse E41 centre (-28.8177, -93.2645) end of major axis (-25.9892, -96.0929) minor radius 1 (-29.5248, -93.9716) -> (-28.1106, -92.5574) ccw
  line L42 (-29.5248, -93.9716) -> (-36.1716, -87.3248)
  ellipse E42 centre (-35.4645, -86.6177) end of major axis (-32.636, -89.4461) minor radius 1 (-34.7574, -85.9106) -> (-36.1716, -87.3248) ccw
  ellipse E43 centre (-73.5355, -93.2645) end of major axis (-70.7071, -90.436) minor radius 1 (-74.2426, -92.5574) -> (-72.8284, -93.9716) ccw
  line L43 (-74.2426, -92.5574) -> (-56.8095, -75.1242)
  ellipse E44 centre (-56.1024, -75.8313) end of major axis (-53.2739, -73.0029) minor radius 1 (-55.3953, -76.5384) -> (-56.8095, -75.1242) ccw
  line L44 (-55.3953, -76.5384) -> (-72.8284, -93.9716)
  ellipse E45 centre (-38.4645, -75.7892) end of major axis (-35.636, -78.6177) minor radius 1 (-37.7574, -75.0821) -> (-39.1716, -76.4963) ccw
  line L45 (-37.7574, -75.0821) -> (-20.2821, -92.5574)
  ellipse E46 centre (-20.9892, -93.2645) end of major axis (-18.1608, -96.0929) minor radius 1 (-21.6963, -93.9716) -> (-20.2821, -92.5574) ccw
  line L46 (-21.6963, -93.9716) -> (-39.1716, -76.4963)
  ellipse E47 centre (-58.5355, -93.9213) end of major axis (-55.7071, -91.0929) minor radius 1 (-57.5048, -94.2952) -> (-58.9094, -92.8906) ccw
  ellipse E48 centre (-57.8787, -93.2645) end of major axis (-55.0503, -90.436) minor radius 1 (-58.9094, -92.8906) -> (-57.5048, -94.2952) ccw
  ellipse E49 centre (-65.7071, -93.2645) end of major axis (-62.8787, -90.436) minor radius 1 (-66.4142, -92.5574) -> (-65, -93.9716) ccw
  line L47 (-66.4142, -92.5574) -> (-59.2426, -85.3858)
  ellipse E50 centre (-58.5355, -86.0929) end of major axis (-55.7071, -83.2645) minor radius 1 (-57.8284, -86.8) -> (-59.2426, -85.3858) ccw
  line L48 (-57.8284, -86.8) -> (-65, -93.9716)
  ellipse E51 centre (-35.6289, -93.7569) end of major axis (-32.8005, -96.5853) minor radius 1 (-35.1707, -92.8062) -> (-36.5796, -94.2151) ccw
  ellipse E52 centre (-36.1213, -93.2645) end of major axis (-33.2929, -96.0929) minor radius 1 (-36.5796, -94.2151) -> (-35.1707, -92.8062) ccw
  line L49 (-93.75, -111.8) -> (-0.25, -111.8)
  line L50 (-0.25, -111.8) -> (-0.25, -0.25)
  line L51 (-0.25, -0.25) -> (-93.75, -0.25)
  line L52 (-93.75, -0.25) -> (-93.75, -111.8)
  circle A0 centre (-5, -5) radius 2
  circle A1 centre (-3.5, -95.55) radius 2
  circle A2 centre (-90.5, -95.55) radius 2
  circle A3 centre (-87.5, -6.5) radius 2
  line L53 (-42.5, -83.8) -> (-42.5, -96.8)
  line L54 (-42.5, -96.8) -> (-51.5, -96.8)
  line L55 (-51.5, -96.8) -> (-51.5, -83.8)
  line L56 (-51.5, -83.8) -> (-42.5, -83.8)
  line L57 (-42, -100.3) -> (-42, -110.3)
  line L58 (-42, -110.3) -> (-43.9689, -110.3)
  line L59 (-43.9689, -110.3) -> (-43.9689, -103.55)
  line L60 (-43.9689, -103.55) -> (-47, -101.8)
  line L61 (-47, -101.8) -> (-50.0311, -103.55)
  line L62 (-50.0311, -103.55) -> (-50.0311, -110.3)
  line L63 (-50.0311, -110.3) -> (-52, -110.3)
  line L64 (-52, -110.3) -> (-52, -100.3)
  line L65 (-52, -100.3) -> (-55, -100.3)
  line L66 (-55, -100.3) -> (-55, -80.3)
  line L67 (-55, -80.3) -> (-52, -80.3)
  line L68 (-52, -80.3) -> (-52, -81.8)
  line L69 (-52, -81.8) -> (-53.5, -81.8)
  line L70 (-53.5, -81.8) -> (-53.5, -98.8)
  line L71 (-53.5, -98.8) -> (-40.5, -98.8)
  line L72 (-40.5, -98.8) -> (-40.5, -81.8)
  line L73 (-40.5, -81.8) -> (-42, -81.8)
  line L74 (-42, -81.8) -> (-42, -80.3)
  line L75 (-42, -80.3) -> (-39, -80.3)
  line L76 (-39, -80.3) -> (-39, -100.3)
  line L77 (-39, -100.3) -> (-42, -100.3)
  line L78 (-5, -5) -> (0, -5)
  line L79 (0, -5) -> (0, 0)
  line L80 (0, 0) -> (-5, 0)
  line L81 (-5, 0) -> (-5, -5)
  line L82 (-87.5, -6.5) -> (-93.75, -6.5)
  line L83 (-93.75, -6.5) -> (-93.75, -0.25)
  line L84 (-93.75, -0.25) -> (-87.5, -0.25)
  line L85 (-87.5, -0.25) -> (-87.5, -6.5)
  line L86 (-93.75, -0.25) -> (-88.75, -0.25)
  line L87 (-88.75, -0.25) -> (-88.75, -4.8699)
  line L88 (-88.75, -4.8699) -> (-93.75, -4.8699)
  line L89 (-93.75, -4.8699) -> (-93.75, -0.25)
  line L90 (-87.5, -6.5) -> (-93.75, -6.5)
  line L91 (-93.75, -6.5) -> (-93.75, -0.25)
  line L92 (-93.75, -0.25) -> (-87.5, -0.25)
  line L93 (-87.5, -0.25) -> (-87.5, -6.5)
  circle A4 centre (-5, -5) radius 2
  circle A5 centre (-87.5, -6.5) radius 2
  dimension "d257" = 5
  dimension "d258" = 4.6199
  constraint horizontal L78
  constraint vertical L79
  constraint horizontal L80
  constraint vertical L81
  constraint coincident L79.end L80.start
  constraint coincident A0.centre L78.start
  constraint horizontal L82
  constraint vertical L83
  constraint horizontal L84
  constraint vertical L85
  constraint coincident L51.end L52.start
  constraint coincident A3.centre L82.start
  constraint horizontal L86
  constraint vertical L87
  constraint horizontal L88
  constraint vertical L89
  constraint horizontal L90
  constraint vertical L91
  constraint horizontal L92
  constraint vertical L93
  constraint concentric A0 A4
  measures "d257" distance of L51.end L86.end
  measures "d258" distance of L51.end L88.end
extrude "Extrude15" add sketch "Sketch11" against normal blind 1.5 contours A3 L82 L85 L90 L93 A5 | A3 L82 L85 L90 L93 A5 | A0 L78 L81 A4 | A0 L78 L81 A4